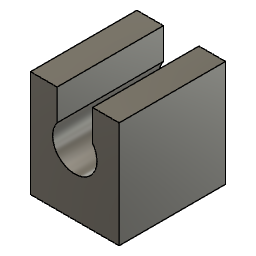
bowden_inside_board_holder (Autodesk Fusion 360 design; units mm, degrees)
Autodesk Fusion 360 part; units mm, degrees
sketch "Sketch1" plane through (0, 0, 0) normal (0, 0, 1) x (1, 0, 0)
  line L0 (0, 0) -> (10, 0)
  line L1 (10, 0) -> (10, 12)
  line L2 (10, 12) -> (0, 12)
  line L3 (0, 12) -> (0, 0)
  line L4 (5, 0) -> (5, 7)
  circle A0 centre (5, 7) radius 2.5
  line L5 (5, 7) -> (7, 7)
  line L6 (7, 7) -> (7, 12)
  line L7 (3, 7) -> (3, 12)
  dimension "d1" = 10
  dimension "d2" = 12
  dimension "d3" = 7
  dimension "d4" = 5
  dimension "d5" = 2
  constraint horizontal L0
  constraint vertical L1
  constraint horizontal L2
  constraint vertical L3
  constraint coincident L0.start L3.end
  constraint midpoint L0 L4.start
  constraint perpendicular L0 L4
  constraint coincident L4.end A0.centre
  constraint perpendicular L4 L5
  constraint coincident L2 L6.end
  constraint perpendicular L2 L6
  constraint symmetric L4 L5.end L7.start
  constraint symmetric L4 L6.end L7.end
  measures "d1" distance of L0.start L0.end
  measures "d2" distance of L0.start L2.end
  measures "d3" distance of L4.start L4.end
  measures "d4" diameter of A0
  measures "d5" distance of L4.end L5.end
extrude "Extrude1" add sketch "Sketch1" along normal blind 12 contours L0 L2 L3 L4 A0 L7 | L0 L1 L2 L4 A0 L6
